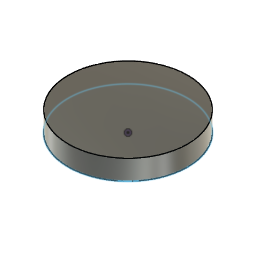
Button Top v4 (Autodesk Fusion 360 design; units mm, degrees)
Autodesk Fusion 360 part; units mm, degrees
sketch "Sketch1" plane through (0, 0, 0) normal (0, 0, 1) x (1, 0, 0)
  circle A0 centre (0, 0) radius 15
  constraint coincident A0.centre origin
extrude "Extrude1" add sketch "Sketch1" along normal blind 5
shell "Shell1" thickness 1 removed faces 1 at (3.8315, 5.6199, 5)
sketch "Sketch2" plane through (0, 0, 1) normal (0, 0, 1) x (-1, 0, 0)
  circle A0 centre (0, 0) radius 14
  circle A1 centre (0, 0) radius 4
  circle A2 centre (0, 0) radius 3.5
  dimension "d4" = 8
  dimension "d5" = 7
  constraint concentric A0 A1
  constraint concentric A0 A2
  measures "d4" diameter of A1
  measures "d5" diameter of A2
extrude "Extrude3" add sketch "Sketch2" along normal blind 6.5 contours A1
extrude "Extrude4" add 1 faces at (-3.8184, 0.1987, 7.5) along direction (0, 0, 1) blind 2
extrude "Extrude5" cut 1 faces at (-3.8184, 0.1987, 9.5) along direction (0, 0, -1) blind 1.5
move_body "Move1" bodies 1 to x (1, 0, 0) y (0, -1, 0) z (0, 0, -1) at (0, 0, 0)
move_body "Move2" bodies 1 to x (1, 0, 0) y (0, 1, 0) z (0, 0, 1) at (0, 0, 5)
